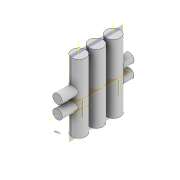
# Autodesk Inventor part: Valves
Saved by Autodesk Inventor 2020 (Build 240168000, 168)
## iProperties
Created: 2019-11-17
Part Number: Valves
Material: Generic
Document SubType Name: Modeling
Designer: ball
Density: 1 g/cm^3
Appearance: Default
Author: ball
Autodesk Inventor part; units mm, degrees
ref_plane "YZ Plane" through (0, 0, 0) normal (1, 0, 0) x (0, 1, 0)
ref_plane "XZ Plane" through (0, 0, 0) normal (0, 1, 0) x (-1, 0, 0)
ref_plane "XY Plane" through (0, 0, 0) normal (0, 0, 1) x (1, 0, 0)
sketch "Sketch1" plane through (0, 0, 0) normal (0, 1, 0) x (-1, 0, 0)
  circle A0 centre (0, 8.5965) radius 9.9822
  circle A1 centre (0, -40.0191) radius 9.9822
  circle A2 centre (0, -15.7113) radius 9.9822
  point P0 (0, 0)
  dimension "d0" = 19.9644
  dimension "d2" = 19.9644
  dimension "d4" = 19.9644
  constraints: 3 centre point
  measures "d0" diameter of A0
  measures "d2" diameter of A1
  measures "d4" diameter of A2
extrude "Extrusion1" add sketch "Sketch1" along normal blind 96.52
ref_plane "Work Plane1" through (0, 48.26, -15.7113) normal (0, 1, 0) x (1, 0, 0)
ref_plane "Work Plane2" through (0, 96.52, 8.5965) normal (-1, 0, 0) x (0, 1, 0)
sketch "Sketch2" plane through (0, 96.52, 8.5965) normal (-1, 0, 0) x (0, 1, 0)
  line L0 (-66.6496, -34.925) -> (-66.6496, 3.175)
  line L1 (-66.6496, 3.175) -> (-34.5694, 3.175)
  line L2 (-34.5694, 3.175) -> (-34.5694, -34.925)
  line L3 (-96.52, -9.9822) -> (-96.52, 9.9822) projected
  line L4 (-34.5694, -34.925) -> (-47.8028, -34.925)
  line L5 (-47.8028, -34.925) -> (-47.8028, -1.5875)
  line L6 (-47.8028, -1.5875) -> (-34.5694, -1.5875)
  line L7 (-34.5694, -1.5875) -> (-34.5694, -34.925)
  line L8 (-66.6496, -34.925) -> (-53.4162, -34.925)
  line L9 (-53.4162, -34.925) -> (-53.4162, 4.7625)
  line L10 (-53.4162, 4.7625) -> (-66.6496, 4.7625)
  line L11 (-66.6496, 4.7625) -> (-66.6496, -34.925)
  line L12 (-34.5694, -34.925) -> (-47.8028, -34.925)
  line L13 (-53.4162, -34.925) -> (-66.6496, -34.925)
  line L14 (-60.0329, -34.925) -> (-60.0329, -4.7625)
  line L15 (-60.0329, -34.925) -> (-29.8704, -34.925) construction
  line L16 (-41.1861, -34.925) -> (-41.1861, -1.5875)
  point P0 (-96.52, 8.5965)
  dimension "d7" = 32.0802
  dimension "d8" = 29.8704
  dimension "d9" = 13.2334
  dimension "d10" = 13.2334
  dimension "d11" = 90
  constraints: 32 end point, 7 parallel, 5 horizontal, 5 perpendicular, 2 midpoint, 1 point on line
  measures "d7" distance of L0.end L1.end
  measures "d8" distance between parallel lines of L3 L0
  measures "d9" distance of L5.end L6.end
  measures "d10" distance of L10.end L9.end
  measures "d11" angle of L15 L14
ref_plane "Work Plane3" through (0, 36.4871, 13.359) normal (0, 1, 0) x (-1, 0, 0)
ref_plane "Work Plane4" through (0, 36.4871, 13.359) normal (0, 0, -1) x (-1, 0, 0)
sketch "Sketch3" plane through (0, 36.4871, 13.359) normal (0, 0, -1) x (-1, 0, 0)
  circle A0 centre (0, 19.8501) radius 6.6167
  circle A1 centre (0, 1.0033) radius 6.6167
  line L0 (9.9822, -36.4871) -> (-9.9822, -36.4871) projected
  point P0 (0, -36.4871)
  dimension "d12" = 13.2334
  dimension "d13" = 13.2334
  dimension "d14" = 18.8468
  dimension "d15" = 37.4904
  constraints: 2 centre point
  measures "d12" diameter of A0
  measures "d13" diameter of A1
  measures "d14" distance of A1.centre A0.centre
  measures "d15" distance from line of L0 A1.centre
extrude "Extrusion2" add sketch "Sketch3" against normal blind 25.4
ref_plane "Work Plane5" through (0, 36.4871, -37.441) normal (0, 0, -1) x (-1, 0, 0)
sketch "Sketch4" plane through (0, 36.4871, -37.441) normal (0, 0, -1) x (-1, 0, 0)
  circle A0 centre (0, 0.7493) radius 6.5024
  line L0 (9.9822, -36.4871) -> (-9.9822, -36.4871) projected
  circle A1 centre (0, 19.4056) radius 6.6421
  point P0 (0, -36.4871)
  dimension "d19" = 13.0048
  dimension "d20" = 37.2364
  dimension "d21" = 13.2842
  dimension "d22" = 18.6563
  constraints: 2 centre point
  measures "d19" diameter of A0
  measures "d20" distance from line of L0 A0.centre
  measures "d21" diameter of A1
  measures "d22" distance of A0.centre A1.centre
extrude "Extrusion3" add sketch "Sketch4" along normal blind 25.4
sketch "Sketch5" plane through (0, 36.4871, 13.359) normal (0, 1, 0) x (-1, 0, 0)
  line L0 (-24.3242, 48.3513) -> (-17.297, 48.3513) construction
  line L1 (-17.297, 48.3513) -> (-17.297, 45.0959) construction
  line L2 (-17.297, 45.0959) -> (-24.3242, 45.0959) construction
  line L3 (-24.3242, 45.0959) -> (-24.3242, 48.3513) construction
  point P0 (0, -13.359)
  constraints: 2 other
body "Solid1"
